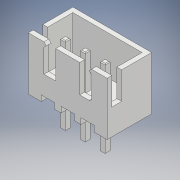
# Autodesk Inventor part: Connecteur jst 3 broches femelle
Saved by Autodesk Inventor 2017 (Build 210142000, 142)
## iProperties
Part Number: Connecteur jst 3 broches femelle
Material: Plastique ABS
Document SubType Name: Modeling
Designer: Adrien MARY
Mass: 0.190573 g
Surface Area: 5.10695 cm^2
Volume: 0.179786 cm^3
Density: 1.06 g/cm^3
Appearance: Lisse - Blanc
Author: Adrien MARY
Autodesk Inventor part; units mm, degrees
ref_plane "YZ Plane" through (0, 0, 0) normal (1, 0, 0) x (0, 1, 0)
ref_plane "XZ Plane" through (0, 0, 0) normal (0, 1, 0) x (-1, 0, 0)
ref_plane "XY Plane" through (0, 0, 0) normal (0, 0, 1) x (1, 0, 0)
sketch "Esquisse1" plane through (0, 0, 0) normal (0, 0, 1) x (1, 0, 0)
  line L0 (-5.04, -2.85) -> (5.04, -2.85)
  line L1 (5.04, -2.85) -> (5.04, 2.85)
  line L2 (5.04, 2.85) -> (-5.04, 2.85)
  line L3 (-5.04, 2.85) -> (-5.04, -2.85)
  line L4 (-5.04, -2.85) -> (5.04, 2.85) construction
  line L5 (5.04, -2.85) -> (-5.04, 2.85) construction
  point P0 (0, 0)
  dimension "Longueur" = 10.08
  dimension "Largueur" = 5.7
  constraints: 12 end point, 2 midpoint, 2 parallel, 1 horizontal, 1 perpendicular
  measures "Longueur" distance of L2.end L1.end
  measures "Largueur" distance of L1.end L0.end
extrude "Embase" add sketch "Esquisse1" along normal mid plane 6.8
shell "Coque1" thickness 0.61 removed faces 1 at (1.68, -0.95, 3.4)
thicken "Epaississement1" operation add thickness 1.19 both sides no extend neighbours yes toward (0, 0, 1) faces at (1.4767, -0.7467, -2.79)
sketch "Esquisse2" plane through (5.04, -2.85, 3.4) normal (1, 0, 0) x (0, 0, -1)
  line L0 (3.5, 0.61) -> (0, 0.61)
  line L1 (0, 0.61) -> (0, 1.86)
  line L2 (0, 1.86) -> (3.5, 1.86)
  line L3 (3.5, 1.86) -> (3.5, 0.61)
  line L4 (0, 0) -> (0, 5.7) projected
  line L5 (6.8, 5.7) -> (0, 5.7) projected
  line L6 (0, 0.61) -> (6.19, 0.61) construction
  point P0 (3.4, 2.85)
  dimension "Profondeur_rainure" = 3.5
  dimension "Largueur_rainure" = 1.25
  constraints: 8 end point, 2 collinear, 2 parallel, 1 horizontal, 1 perpendicular
  measures "Profondeur_rainure" distance of L1.end L2.end
  measures "Largueur_rainure" distance of L0.end L1.end
extrude "Rainure" cut sketch "Esquisse2" against normal through all
sketch "Esquisse3" plane through (-5.04, -2.85, 3.4) normal (0, -1, 0) x (1, 0, 0)
  line L0 (2.54, 0) -> (2.84, -0.3)
  line L1 (2.84, -0.3) -> (2.54, -0.6)
  line L2 (2.54, -0.6) -> (2.54, -3.6)
  line L3 (2.54, -3.6) -> (7.54, -3.6)
  line L4 (7.54, -3.6) -> (7.54, -0.6)
  line L5 (7.54, -0.6) -> (7.24, -0.3)
  line L6 (7.24, -0.3) -> (7.54, 0)
  line L7 (7.54, 0) -> (2.54, 0)
  line L8 (0, 0) -> (10.08, 0) projected
  point P0 (5.04, -3.4)
  point P1 (5.04, 0)
  point P2 (5.04, -3.6)
  dimension "Profondeur_ouverture" = 3.6
  dimension "Largueur_ouverture" = 5
  dimension "d12" = 0.3
  constraints: 16 end point, 6 perpendicular, 2 midpoint, 2 vertical alignment, 1 collinear, 1 horizontal alignment, 1 parallel, 1 point on line, 1 vertical
  measures "Profondeur_ouverture" distance between parallel lines of L7 L3
  measures "Largueur_ouverture" distance of L2.end L3.end
  measures "d12" distance from line of L7 L0.end
extrude "Ouverture_avant_2_broches" [suppressed]
fillet "Congé1" [suppressed]
ref_plane "Plan de construction3" through (2.54, -2.85, -3.4) normal (1, 0, 0) x (0, 0, -1)
sketch "Esquisse6" plane through (2.54, -2.85, -3.4) normal (1, 0, 0) x (0, 0, -1)
  line L0 (-0.75, 0) -> (-0.125, 1.65)
  line L1 (-0.125, 1.65) -> (-0.125, 2.85)
  line L2 (-0.125, 2.85) -> (-0.75, 5.7)
  line L3 (-0.75, 5.7) -> (0, 5.7)
  line L4 (0, 5.7) -> (0, 0)
  line L5 (0, 0) -> (-0.75, 0)
  line L6 (-6.8, 0.61) -> (-3.3, 0.61) construction
  line L7 (-3.3, 0.61) -> (-3.3, 1.86) construction
  line L8 (-3.3, 1.86) -> (-6.8, 1.86) construction
  line L9 (-6.8, 5.7) -> (-6.8, 1.86) construction
  line L10 (0, 5.7) -> (-6.8, 5.7) construction
  line L11 (0, 0) -> (0, 5.7) construction
  line L12 (-6.8, 0) -> (0, 0) construction
  line L13 (-6.8, 0.61) -> (-6.8, 0) construction
  point P0 (-3.4, 2.85)
  dimension "d36" = 0.125
  dimension "d37" = 0.75
  dimension "d38" = 1.65
  dimension "d39" = 2.85
  constraints: 12 end point, 3 collinear, 2 perpendicular, 1 vertical, 1 vertical alignment
  measures "d36" distance between parallel lines of L4 L1
  measures "d37" distance of L2.end L3.end
  measures "d38" vertical distance of L0.start L0.end
  measures "d39" vertical distance of L1.end L2.end
extrude "Extrusion6" cut sketch "Esquisse6" along normal mid plane 1.7
sketch "Esquisse7" plane through (2.54, -2.85, -3.4) normal (1, 0, 0) x (0, 0, -1)
  line L0 (3.7, 1.925) -> (-6.3, 1.925)
  line L1 (-6.3, 1.925) -> (-6.3, 2.575)
  line L2 (-6.3, 2.575) -> (3.7, 2.575)
  line L3 (3.7, 2.575) -> (3.7, 1.925)
  line L4 (-1.8, 0.61) -> (-1.8, 5.09) projected
  line L5 (-0.125, 1.65) -> (-0.125, 2.85) construction
  point P0 (-3.4, 2.85)
  point P1 (-6.3, 2.25)
  point P2 (-0.125, 2.25)
  dimension "Hauteur_broche" = 10
  dimension "d43" = 0.65
  dimension "d44" = 4.5
  constraints: 8 end point, 2 midpoint, 2 parallel, 1 horizontal, 1 horizontal alignment, 1 perpendicular
  measures "Hauteur_broche" distance of L1.end L2.end
  measures "d43" distance of L0.end L1.end
  measures "d44" distance between parallel lines of L4 L1
extrude "Extrusion7" add sketch "Esquisse7" along normal mid plane 0.63
chamfer "Chanfrein2" distance 0.1 angle 45 8 edges at (2.855, -0.6, 2.9) (2.54, -0.925, 2.9) (2.225, -0.6, 2.9) (2.54, -0.275, 2.9) (2.54, -0.925, -7.1) (2.855, -0.6, -7.1) (2.54, -0.275, -7.1) (2.225, -0.6, -7.1)
pattern_linear "Réseau rectangulaire1" count 3 spacing 2.54 along (-1, 0, 0) of "Extrusion6", "Extrusion7", "Chanfrein2"
sketch "Esquisse8" plane through (5.04, -2.85, -3.4) normal (0, -1, 0) x (1, 0, 0)
  line L0 (-3.5, 6.8) -> (-2, 6.8)
  line L1 (-2, 6.2) -> (-2, 3.2)
  line L2 (-2, 3.2) -> (-3.5, 3.2)
  line L3 (-3.5, 3.2) -> (-3.5, 6.8)
  line L4 (-10.08, 6.8) -> (0, 6.8) projected
  line L5 (0, 0) -> (0, 6.8) projected
  line L6 (-2, 6.2) -> (-2.3, 6.5)
  line L7 (-2.3, 6.5) -> (-2, 6.8)
  point P0 (-5.04, 3.4)
  point P1 (-1.27, 6.8)
  dimension "d53" = 2
  dimension "d54" = 1.5
  dimension "d55" = 3.6
  dimension "d56" = 0.3
  dimension "d57" = 90
  constraints: 12 end point, 2 parallel, 2 perpendicular, 1 collinear, 1 horizontal, 1 vertical alignment
  measures "d53" distance between parallel lines of L5 L1
  measures "d54" distance of L1.end L2.end
  measures "d55" distance of L0.end L1.end
  measures "d56" distance from line of L0 L6.end
  measures "d57" angle of L6 L7
extrude "Ouverture avant sup a2 broches" cut sketch "Esquisse8" against normal up to surface (0.61 mm away)
fillet "Congé2" radius 0.3 1 edges at (3.04, -2.545, -0.2)
mirror "Symétrie2" about plane through (0, 0, 0) normal (1, 0, 0) of "Ouverture avant sup a2 broches"
